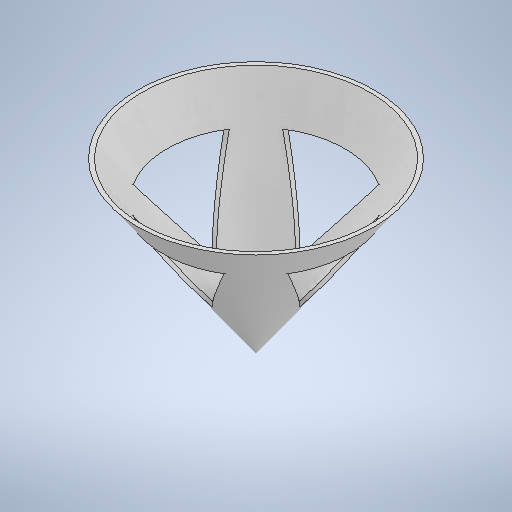
# Autodesk Inventor part: small_membrane_shell
Saved by Autodesk Inventor 2025.2 (Build 292293000, 293)
## iProperties
Created: 2025-03-05
Part Number: small_membrane_shell
Material: Generic
Document SubType Name: Modeling
Designer: fiste
Density: 1 g/cm^3
Appearance: Default
Author: fiste
Autodesk Inventor part; units mm, degrees
ref_plane "YZ Plane" through (0, 0, 0) normal (1, 0, 0) x (0, 1, 0)
ref_plane "XZ Plane" through (0, 0, 0) normal (0, 1, 0) x (-1, 0, 0)
ref_plane "XY Plane" through (0, 0, 0) normal (0, 0, 1) x (1, 0, 0)
sketch "Sketch1" plane through (0, 0, 0) normal (0, 1, 0) x (-1, 0, 0)
  line L0 (38, 0) -> (0, -54.2696)
  line L1 (38, 0) -> (104.251, 0) construction
  line L2 (0, -54.2696) -> (0, -56.2696)
  line L3 (0, -56.2696) -> (39.4004, 0)
  line L4 (39.4004, 0) -> (38, 0)
  line L5 (0, -67.5235) -> (0, 11.2539) projected
  point P0 (0, 0)
  dimension "d0" = 125
  dimension "d1" = 2
  constraints: 10 end point, 1 equal length, 1 horizontal, 1 parallel, 1 perpendicular, 1 vertical
  measures "d0" angle of L0 L1
  measures "d1" distance of L0.end L2.end
revolve "Revolution1" add sketch "Sketch1" angle 360 about axis through (0, 0, -10) along (0, 0, 1)
sketch "Sketch3" plane through (0, 0, 0) normal (0, 1, 0) x (-1, 0, 0)
  line L0 (16, -12) -> (-16, -12)
  line L1 (-16, -12) -> (0, -35.4925)
  line L2 (0, -35.4925) -> (16, -12)
  point P0 (0, 0)
  dimension "d3" = 32
  constraints: 6 end point, 1 horizontal
  measures "d3" distance of L0.start L0.end
extrude "Extrusion1" cut sketch "Sketch3" along normal mid plane 70
pattern_circular "Circular Pattern1" count 2 over 90 about axis through (0, 0, -10) along (0, 0, 1) of "Extrusion1"
body "Solid1"
